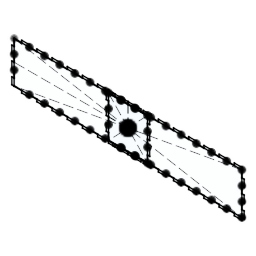
MVP (Autodesk Fusion 360 design; units mm, degrees)
part number: 2026-03-07-18-20-50-739
Autodesk Fusion 360 part; units mm, degrees
sketch "Front" plane through (0, 0, 0) normal (0, 0, 1) x (1, 0, 0)
  line L0 (132, 16) -> (-132, 16)
  line L1 (-132, 16) -> (-132, -16)
  line L2 (-132, -16) -> (132, -16)
  line L3 (132, -16) -> (132, 16)
  line L4 (132, 16) -> (-132, -16) construction
  line L5 (-132, 16) -> (132, -16) construction
  line L6 (152, 26) -> (-152, 26)
  line L7 (-152, 26) -> (-152, -26)
  line L8 (-152, -26) -> (152, -26)
  line L9 (152, -26) -> (152, 26)
  line L10 (152, 26) -> (-152, -26) construction
  line L11 (-152, 26) -> (152, -26) construction
  line L12 (0, 0) -> (0, -16) construction
  line L13 (0, 0) -> (12, 0) construction
  line L14 (0, 0) -> (-132, 0) construction
  line L15 (-132, 0) -> (-132, -19) construction
  line L16 (-132, -19) -> (-136, -19) construction
  line L17 (-136, -19) -> (-148, -19) construction
  line L18 (-142, -19) -> (-142, -14.5) construction
  circle A0 centre (-142, -14.5) radius 1.5
  circle A1 centre (-142, 14.5) radius 1.5
  circle A2 centre (142, 14.5) radius 1.5
  circle A3 centre (142, -14.5) radius 1.5
  line L19 (-152, 26) -> (-152, 29)
  line L20 (-152, 29) -> (-141.8667, 29)
  line L21 (-141.8667, 29) -> (-141.8667, 26)
  line L22 (-141.8667, 26) -> (-131.7333, 26)
  line L23 (-121.6, 29) -> (-121.6, 26)
  line L24 (-121.6, 26) -> (-111.4667, 26)
  line L25 (-131.7333, 29) -> (-121.6, 29)
  line L26 (-131.7333, 26) -> (-131.7333, 29)
  line L27 (-101.3333, 29) -> (-101.3333, 26)
  line L28 (-101.3333, 26) -> (-91.2, 26)
  line L29 (-111.4667, 29) -> (-101.3333, 29)
  line L30 (-111.4667, 26) -> (-111.4667, 29)
  line L31 (-81.0667, 29) -> (-81.0667, 26)
  line L32 (-81.0667, 26) -> (-70.9333, 26)
  line L33 (-91.2, 29) -> (-81.0667, 29)
  line L34 (-91.2, 26) -> (-91.2, 29)
  line L35 (-60.8, 29) -> (-60.8, 26)
  line L36 (-60.8, 26) -> (-50.6667, 26)
  line L37 (-70.9333, 29) -> (-60.8, 29)
  line L38 (-70.9333, 26) -> (-70.9333, 29)
  line L39 (-40.5333, 29) -> (-40.5333, 26)
  line L40 (-40.5333, 26) -> (-30.4, 26)
  line L41 (-50.6667, 29) -> (-40.5333, 29)
  line L42 (-50.6667, 26) -> (-50.6667, 29)
  line L43 (-20.2667, 29) -> (-20.2667, 26)
  line L44 (-20.2667, 26) -> (-10.1333, 26)
  line L45 (-30.4, 29) -> (-20.2667, 29)
  line L46 (-30.4, 26) -> (-30.4, 29)
  line L47 (0, 29) -> (0, 26)
  line L48 (0, 26) -> (10.1333, 26)
  line L49 (-10.1333, 29) -> (0, 29)
  line L50 (-10.1333, 26) -> (-10.1333, 29)
  line L51 (20.2667, 29) -> (20.2667, 26)
  line L52 (20.2667, 26) -> (30.4, 26)
  line L53 (10.1333, 29) -> (20.2667, 29)
  line L54 (10.1333, 26) -> (10.1333, 29)
  line L55 (40.5333, 29) -> (40.5333, 26)
  line L56 (40.5333, 26) -> (50.6667, 26)
  line L57 (30.4, 29) -> (40.5333, 29)
  line L58 (30.4, 26) -> (30.4, 29)
  line L59 (60.8, 29) -> (60.8, 26)
  line L60 (60.8, 26) -> (70.9333, 26)
  line L61 (50.6667, 29) -> (60.8, 29)
  line L62 (50.6667, 26) -> (50.6667, 29)
  line L63 (81.0667, 29) -> (81.0667, 26)
  line L64 (81.0667, 26) -> (91.2, 26)
  line L65 (70.9333, 29) -> (81.0667, 29)
  line L66 (70.9333, 26) -> (70.9333, 29)
  line L67 (101.3333, 29) -> (101.3333, 26)
  line L68 (101.3333, 26) -> (111.4667, 26)
  line L69 (91.2, 29) -> (101.3333, 29)
  line L70 (91.2, 26) -> (91.2, 29)
  line L71 (121.6, 29) -> (121.6, 26)
  line L72 (121.6, 26) -> (131.7333, 26)
  line L73 (111.4667, 29) -> (121.6, 29)
  line L74 (111.4667, 26) -> (111.4667, 29)
  line L75 (141.8667, 29) -> (141.8667, 26)
  line L76 (141.8667, 26) -> (152, 26)
  line L77 (131.7333, 29) -> (141.8667, 29)
  line L78 (131.7333, 26) -> (131.7333, 29)
  line L79 (-152, -26) -> (-152, -29)
  line L80 (-152, -29) -> (-141.8667, -29)
  line L81 (-141.8667, -29) -> (-141.8667, -26)
  line L82 (-141.8667, -26) -> (-131.7333, -26)
  line L83 (-131.7333, -26) -> (-131.7333, -29)
  line L84 (-131.7333, -29) -> (-121.6, -29)
  line L85 (-121.6, -29) -> (-121.6, -26)
  line L86 (-121.6, -26) -> (-111.4667, -26)
  line L87 (-111.4667, -26) -> (-111.4667, -29)
  line L88 (-111.4667, -29) -> (-101.3333, -29)
  line L89 (-101.3333, -29) -> (-101.3333, -26)
  line L90 (-101.3333, -26) -> (-91.2, -26)
  line L91 (-91.2, -26) -> (-91.2, -29)
  line L92 (-91.2, -29) -> (-81.0667, -29)
  line L93 (-81.0667, -29) -> (-81.0667, -26)
  line L94 (-81.0667, -26) -> (-70.9333, -26)
  line L95 (-70.9333, -26) -> (-70.9333, -29)
  line L96 (-70.9333, -29) -> (-60.8, -29)
  line L97 (-60.8, -29) -> (-60.8, -26)
  line L98 (-60.8, -26) -> (-50.6667, -26)
  line L99 (-50.6667, -26) -> (-50.6667, -29)
  line L100 (-50.6667, -29) -> (-40.5333, -29)
  line L101 (-40.5333, -29) -> (-40.5333, -26)
  line L102 (-40.5333, -26) -> (-30.4, -26)
  line L103 (-30.4, -26) -> (-30.4, -29)
  line L104 (-30.4, -29) -> (-20.2667, -29)
  line L105 (-20.2667, -29) -> (-20.2667, -26)
  line L106 (-20.2667, -26) -> (-10.1333, -26)
  line L107 (-10.1333, -26) -> (-10.1333, -29)
  line L108 (-10.1333, -29) -> (0, -29)
  line L109 (0, -29) -> (0, -26)
  line L110 (0, -26) -> (10.1333, -26)
  line L111 (10.1333, -26) -> (10.1333, -29)
  line L112 (10.1333, -29) -> (20.2667, -29)
  line L113 (20.2667, -29) -> (20.2667, -26)
  line L114 (20.2667, -26) -> (30.4, -26)
  line L115 (30.4, -26) -> (30.4, -29)
  line L116 (30.4, -29) -> (40.5333, -29)
  line L117 (40.5333, -29) -> (40.5333, -26)
  line L118 (40.5333, -26) -> (50.6667, -26)
  line L119 (50.6667, -26) -> (50.6667, -29)
  line L120 (50.6667, -29) -> (60.8, -29)
  line L121 (60.8, -29) -> (60.8, -26)
  line L122 (60.8, -26) -> (70.9333, -26)
  line L123 (70.9333, -26) -> (70.9333, -29)
  line L124 (70.9333, -29) -> (81.0667, -29)
  line L125 (81.0667, -29) -> (81.0667, -26)
  line L126 (81.0667, -26) -> (91.2, -26)
  line L127 (91.2, -26) -> (91.2, -29)
  line L128 (91.2, -29) -> (101.3333, -29)
  line L129 (101.3333, -29) -> (101.3333, -26)
  line L130 (101.3333, -26) -> (111.4667, -26)
  line L131 (111.4667, -26) -> (111.4667, -29)
  line L132 (111.4667, -29) -> (121.6, -29)
  line L133 (121.6, -29) -> (121.6, -26)
  line L134 (121.6, -26) -> (131.7333, -26)
  line L135 (131.7333, -26) -> (131.7333, -29)
  line L136 (131.7333, -29) -> (141.8667, -29)
  line L137 (141.8667, -29) -> (141.8667, -26)
  line L138 (141.8667, -26) -> (152, -26)
  line L139 (-152, -26) -> (-152, -17.3333)
  line L140 (-152, -17.3333) -> (-155, -17.3333)
  line L141 (-155, -17.3333) -> (-155, -8.6667)
  line L142 (-155, -8.6667) -> (-152, -8.6667)
  line L143 (-155, 0) -> (-155, 8.6667)
  line L144 (-152, 0) -> (-155, 0)
  line L145 (-155, 8.6667) -> (-152, 8.6667)
  line L146 (-152, -8.6667) -> (-152, 0)
  line L147 (-155, 17.3333) -> (-155, 26)
  line L148 (-152, 17.3333) -> (-155, 17.3333)
  line L149 (-155, 26) -> (-152, 26)
  line L150 (-152, 8.6667) -> (-152, 17.3333)
  line L151 (155, 17.3333) -> (155, 26)
  line L152 (152, 17.3333) -> (155, 17.3333)
  line L153 (152, 8.6667) -> (152, 17.3333)
  line L154 (155, 26) -> (152, 26)
  line L155 (155, 8.6667) -> (152, 8.6667)
  line L156 (155, 0) -> (155, 8.6667)
  line L157 (152, 0) -> (155, 0)
  line L158 (152, -8.6667) -> (152, 0)
  line L159 (155, -17.3333) -> (155, -8.6667)
  line L160 (152, -17.3333) -> (155, -17.3333)
  line L161 (152, -26) -> (152, -17.3333)
  line L162 (155, -8.6667) -> (152, -8.6667)
  dimension "d15" = 264
  dimension "d16" = 32
  dimension "d17" = 304
  dimension "d18" = 52
  dimension "d58" = 16
  dimension "d63" = 12
  dimension "d71" = 132
  dimension "d72" = 19
  dimension "d73" = 4
  dimension "d74" = 12
  dimension "d75" = 4.5
  dimension "d76" = 3
  dimension "d86" = 3
  dimension "d87" = 10.1333
  dimension "d88" = 3
  dimension "d89" = 10.1333
  dimension "d92" = 283.7333
  dimension "d93" = 0
  dimension "d94" = 3
  dimension "d95" = 10.1333
  dimension "d96" = 3
  dimension "d97" = 10.1333
  dimension "d100" = 283.7333
  dimension "d101" = 0
  dimension "d105" = 8.6667
  dimension "d106" = 3
  dimension "d107" = 8.6667
  dimension "d108" = 3
  dimension "d111" = 0
  dimension "d112" = 34.6667
  constraint horizontal L0
  constraint perpendicular L0 L1
  constraint parallel L0 L2
  constraint parallel L1 L3
  constraint coincident L4 L12.start
  constraint coincident L5 L12.start
  constraint coincident L12.start L13.start
  constraint horizontal L6
  constraint perpendicular L6 L7
  constraint parallel L6 L8
  constraint parallel L7 L9
  constraint coincident L10 L12.start
  constraint coincident L11 L12.start
  constraint perpendicular L2 L12
  constraint horizontal L13
  constraint parallel L0 L14
  constraint perpendicular L2 L15
  constraint perpendicular L15 L16
  constraint parallel L16 L17
  constraint midpoint L17 L18.start
  constraint perpendicular L17 L18
  constraint coincident L18.end A0.centre
  constraint symmetric L14 A0 A1
  constraint symmetric L12 A0 A3
  constraint symmetric L12 A1 A2
  constraint perpendicular L6 L19
  constraint perpendicular L19 L20
  constraint perpendicular L20 L21
  constraint perpendicular L21 L22
  constraint perpendicular L8 L79
  constraint perpendicular L79 L80
  constraint perpendicular L8 L81
  constraint perpendicular L81 L82
  constraint perpendicular L8 L139
  constraint perpendicular L7 L140
  constraint perpendicular L140 L141
  constraint coincident L7 L142.end
  constraint perpendicular L7 L142
  constraint symmetric L7.end L12 L8.end
  constraint symmetric L12 L139.end L160.start
  constraint symmetric L12 L140.end L159.start
  constraint symmetric L12 L141.end L159.end
  constraint symmetric L12 L142.end L158.start
  constraint symmetric L12 L143.start L156.start
  constraint symmetric L12 L143.end L155.start
  constraint symmetric L12 L144.start L157.start
  constraint symmetric L12 L145.end L153.start
  constraint symmetric L12 L147.start L151.start
  constraint symmetric L12 L147.end L151.end
  constraint symmetric L12 L148.start L152.start
  constraint symmetric L12 L6.end L6.start
  measures "d15" distance of L1.end L2.end
  measures "d16" distance of L0.end L1.end
  measures "d17" distance of L7.end L8.end
  measures "d18" distance of L6.end L7.end
  measures "d58" distance of L12.start L12.end
  measures "d63" distance of L12.start L13.end
  measures "d71" distance of L12.start L14.end
  measures "d72" distance of L14.end L15.end
  measures "d73" distance of L15.end L16.end
  measures "d74" distance of L16.end L17.end
  measures "d75" distance of L18.start L18.end
  measures "d76" diameter of A0
  measures "d86" distance of L6.end L19.end
  measures "d87" distance of L19.end L20.end
  measures "d88" distance of L20.end L21.end
  measures "d89" distance of L21.end L22.end
  measures "d94" distance of L7.end L79.end
  measures "d95" distance of L79.end L80.end
  measures "d96" distance of L80.end L81.end
  measures "d97" distance of L81.end L82.end
  measures "d105" distance of L7.end L139.end
  measures "d106" distance of L139.end L140.end
  measures "d107" distance of L140.end L141.end
  measures "d108" distance of L141.end L142.end
sketch "Clamp base" plane through (0, 0, 0) normal (0, 0, 1) x (1, 0, 0)
  line L0 (6, 19) -> (-6, 19)
  line L1 (-6, 19) -> (-6, -19)
  line L2 (-6, -19) -> (6, -19)
  line L3 (6, -19) -> (6, 19)
  line L4 (6, 19) -> (-6, -19) construction
  line L5 (-6, 19) -> (6, -19) construction
  line L6 (0, 19) -> (0, 14.5) construction
  circle A0 centre (0, 14.5) radius 1.5
  line L7 (0, 0) -> (6, 0) construction
  circle A1 centre (0, -14.5) radius 1.5
  line L8 (0, -19) -> (0, -14.5) construction
  line L9 (6, 19) -> (9, 19)
  line L10 (9, 19) -> (9, -19)
  line L11 (9, -19) -> (6, -19)
  line L12 (6, -19) -> (6, 19)
  line L13 (6, 19) -> (6, 10) construction
  line L14 (6, 10) -> (-6, 10)
  line L15 (6, -10) -> (-6, -10)
  dimension "d19" = 12
  dimension "d20" = 38
  dimension "d21" = 4.5
  dimension "d22" = 3
  dimension "d23" = 3
  dimension "d24" = 38
  dimension "d67" = 9
  dimension "d68" = 12
  constraint horizontal L0
  constraint perpendicular L0 L1
  constraint parallel L0 L2
  constraint parallel L1 L3
  constraint coincident L4 L7.start
  constraint coincident L5 L7.start
  constraint coincident L7.start origin
  constraint midpoint L0 L6.start
  constraint perpendicular L0 L6
  constraint coincident L6.end A0.centre
  constraint midpoint L3 L7.end
  constraint symmetric L6.start L7 L8.start
  constraint symmetric L6.end L7 A1.centre
  constraint symmetric A0 L7 A1
  constraint horizontal L9
  constraint vertical L10
  constraint horizontal L11
  constraint vertical L12
  constraint perpendicular L0 L13
  constraint perpendicular L1 L14
  constraint symmetric L7 L13.end L15.start
  constraint symmetric L7 L14.end L15.end
  measures "d19" distance of L1.end L2.end
  measures "d20" distance of L0.end L1.end
  measures "d21" distance of L6.start L6.end
  measures "d22" diameter of A0
  measures "d23" distance of L0.start L9.end
  measures "d24" distance of L0.start L2.end
  measures "d67" distance of L0.start L13.end
  measures "d68" distance of L13.end L14.end
extrude "Extrude3" add sketch "Clamp base" along normal blind 2 contours L0 L1 L3 L12 L14 | L1 L3 L12 L14 L15 | L1 L2 L3 L12 L15
extrude "Extrude4" add sketch "Clamp base" along normal blind 11.5 contours L3 L9 L10 L11 L12
sketch "Clamp support wall" plane through (9, 0, 0) normal (1, 0, 0) x (0, 0, -1)
  line L0 (0, -19) -> (0, 19)
  line L1 (0, 19) -> (-11.5, 19)
  line L2 (-11.5, 19) -> (-11.5, -19)
  line L3 (-11.5, -19) -> (0, -19)
  line L4 (-11.5, 19) -> (-5.75, 19) construction
  line L5 (-5.75, 19) -> (-5.75, 17) construction
  line L6 (0, 0) -> (-2, 0) construction
  line L7 (-11.5, 19) -> (-6.1, 19)
  line L8 (-11.5, 19) -> (-6.1, 19)
  line L9 (-6.1, 19) -> (-6.1, 7)
  line L10 (-6.1, 7) -> (-11.5, 7)
  line L11 (-11.5, 7) -> (-11.5, 19)
  line L12 (-6.1, -7) -> (-11.5, -7)
  line L13 (-11.5, -7) -> (-11.5, -19)
  line L14 (-11.5, -19) -> (-6.1, -19)
  line L15 (-6.1, -19) -> (-6.1, -7)
  line L16 (0, 19) -> (0, 10) construction
  line L17 (0, 10) -> (-6.1, 10)
  line L18 (0, -10) -> (-6.1, -10)
  line L19 (-6.1, 7) -> (-6.1, -7)
  dimension "d42" = 2
  dimension "d43" = 2
  dimension "d44" = 5.4
  dimension "d45" = 5.4
  dimension "d46" = 12
  dimension "d77" = 9
  constraint coincident L1.end L2.start
  constraint midpoint L1 L4.end
  constraint perpendicular L1 L5
  constraint coincident L6.start origin
  constraint perpendicular L0 L6
  constraint perpendicular L5 L7
  constraint horizontal L8
  constraint vertical L9
  constraint horizontal L10
  constraint vertical L11
  constraint symmetric L6 L1.end L2.end
  constraint symmetric L6 L7.end L14.end
  constraint symmetric L6 L9.end L12.start
  constraint symmetric L6 L10.end L12.end
  constraint coincident L0.end L1.start
  constraint perpendicular L1 L16
  constraint coincident L9 L17.end
  constraint perpendicular L9 L17
  constraint symmetric L6 L16.end L18.start
  constraint symmetric L6 L17.end L18.end
  measures "d42" distance of L4.end L5.end
  measures "d43" distance of L6.start L6.end
  measures "d44" distance of L1.end L7.end
  measures "d45" distance of L1.end L7.end
  measures "d46" distance of L1.end L10.end
  measures "d77" distance of L0.end L16.end
extrude "Extrude5" add sketch "Clamp support wall" along normal blind 5 contours L2 L3 L12 L13 L14 L15 | L1 L2 L7 L8 L9 L10 L11
sketch "Clamp grooves" plane through (14, 0, 0) normal (1, 0, 0) x (0, 0, -1)
  line L0 (-11.5, 7) -> (-6.1, 7)
  line L1 (-6.1, 7) -> (-6.1, 19)
  line L2 (-6.1, 19) -> (-11.5, 19)
  line L3 (-11.5, 19) -> (-11.5, 7)
  line L4 (0, 0) -> (-2, 0) construction
  line L5 (-6.1, 7) -> (-8.1, 7)
  line L6 (-8.1, 7) -> (-8.1, 17)
  line L7 (-8.1, 17) -> (-9.5, 17)
  line L8 (-9.5, 17) -> (-9.5, 7)
  line L9 (-8.1, -7) -> (-8.1, -17)
  line L10 (-8.1, -17) -> (-9.5, -17)
  line L11 (-9.5, -17) -> (-9.5, -7)
  line L12 (-9.5, 7) -> (-8.1, 7)
  line L13 (-8.1, -7) -> (-9.5, -7)
  dimension "d49" = 2
  dimension "d50" = 2
  dimension "d51" = 10
  dimension "d52" = 1.4
  dimension "d53" = 10
  constraint coincident L4.start origin
  constraint horizontal L4
  constraint coincident L0.end L1.start
  constraint coincident L0 L5.end
  constraint perpendicular L0 L6
  constraint perpendicular L6 L7
  constraint perpendicular L0 L8
  constraint symmetric L4 L5.end L9.start
  constraint symmetric L4 L6.end L9.end
  constraint symmetric L4 L7.end L10.end
  constraint symmetric L4 L8.end L11.end
  measures "d49" distance of L4.start L4.end
  measures "d50" distance of L0.end L5.end
  measures "d51" distance of L5.end L6.end
  measures "d52" distance of L6.end L7.end
  measures "d53" distance of L7.end L8.end
extrude "Extrude8" cut sketch "Clamp grooves" against normal blind 5 contours L0 L6 L7 L8 L12 | L9 L10 L11 L13
extrude "Extrude9" cut sketch "Clamp base" along normal blind 2 contours L1 L3 L12 L14 L15
extrude "Extrude10" cut sketch "Clamp support wall" against normal blind 3 contours L0 L9 L15 L17 L18 L19
sketch "Back" plane through (0, 0, 0) normal (0, 0, 1) x (1, 0, 0)
  line L0 (152, 26) -> (-152, 26)
  line L1 (-152, 26) -> (-152, -26)
  line L2 (-152, -26) -> (152, -26)
  line L3 (152, -26) -> (152, 26)
  line L4 (152, 26) -> (-152, -26) construction
  line L5 (-152, 26) -> (152, -26) construction
  line L6 (0, 0) -> (0, 26) construction
  line L7 (0, 0) -> (-152, 0) construction
  line L8 (-152, 26) -> (-152, 29)
  line L9 (-152, 29) -> (-141.8667, 29)
  line L10 (-141.8667, 29) -> (-141.8667, 26)
  line L11 (-141.8667, 26) -> (-131.7333, 26)
  line L12 (-131.7333, 29) -> (-121.6, 29)
  line L13 (-121.6, 29) -> (-121.6, 26)
  line L14 (-121.6, 26) -> (-111.4667, 26)
  line L15 (-131.7333, 26) -> (-131.7333, 29)
  line L16 (-111.4667, 29) -> (-101.3333, 29)
  line L17 (-101.3333, 29) -> (-101.3333, 26)
  line L18 (-101.3333, 26) -> (-91.2, 26)
  line L19 (-111.4667, 26) -> (-111.4667, 29)
  line L20 (-91.2, 29) -> (-81.0667, 29)
  line L21 (-81.0667, 29) -> (-81.0667, 26)
  line L22 (-81.0667, 26) -> (-70.9333, 26)
  line L23 (-91.2, 26) -> (-91.2, 29)
  line L24 (-70.9333, 29) -> (-60.8, 29)
  line L25 (-60.8, 29) -> (-60.8, 26)
  line L26 (-60.8, 26) -> (-50.6667, 26)
  line L27 (-70.9333, 26) -> (-70.9333, 29)
  line L28 (-50.6667, 29) -> (-40.5333, 29)
  line L29 (-40.5333, 29) -> (-40.5333, 26)
  line L30 (-40.5333, 26) -> (-30.4, 26)
  line L31 (-50.6667, 26) -> (-50.6667, 29)
  line L32 (-30.4, 29) -> (-20.2667, 29)
  line L33 (-20.2667, 29) -> (-20.2667, 26)
  line L34 (-20.2667, 26) -> (-10.1333, 26)
  line L35 (-30.4, 26) -> (-30.4, 29)
  line L36 (-10.1333, 29) -> (0, 29)
  line L37 (0, 29) -> (0, 26)
  line L38 (0, 26) -> (10.1333, 26)
  line L39 (-10.1333, 26) -> (-10.1333, 29)
  line L40 (10.1333, 29) -> (20.2667, 29)
  line L41 (20.2667, 29) -> (20.2667, 26)
  line L42 (20.2667, 26) -> (30.4, 26)
  line L43 (10.1333, 26) -> (10.1333, 29)
  line L44 (30.4, 29) -> (40.5333, 29)
  line L45 (40.5333, 29) -> (40.5333, 26)
  line L46 (40.5333, 26) -> (50.6667, 26)
  line L47 (30.4, 26) -> (30.4, 29)
  line L48 (50.6667, 29) -> (60.8, 29)
  line L49 (60.8, 29) -> (60.8, 26)
  line L50 (60.8, 26) -> (70.9333, 26)
  line L51 (50.6667, 26) -> (50.6667, 29)
  line L52 (70.9333, 29) -> (81.0667, 29)
  line L53 (81.0667, 29) -> (81.0667, 26)
  line L54 (81.0667, 26) -> (91.2, 26)
  line L55 (70.9333, 26) -> (70.9333, 29)
  line L56 (91.2, 29) -> (101.3333, 29)
  line L57 (101.3333, 29) -> (101.3333, 26)
  line L58 (101.3333, 26) -> (111.4667, 26)
  line L59 (91.2, 26) -> (91.2, 29)
  line L60 (111.4667, 29) -> (121.6, 29)
  line L61 (121.6, 29) -> (121.6, 26)
  line L62 (121.6, 26) -> (131.7333, 26)
  line L63 (111.4667, 26) -> (111.4667, 29)
  line L64 (131.7333, 29) -> (141.8667, 29)
  line L65 (141.8667, 29) -> (141.8667, 26)
  line L66 (141.8667, 26) -> (152, 26)
  line L67 (131.7333, 26) -> (131.7333, 29)
  line L68 (-152, -29) -> (-141.8667, -29)
  line L69 (-141.8667, -29) -> (-141.8667, -26)
  line L70 (-141.8667, -26) -> (-131.7333, -26)
  line L71 (-152, -26) -> (-152, -29)
  line L72 (-131.7333, -29) -> (-121.6, -29)
  line L73 (-131.7333, -26) -> (-131.7333, -29)
  line L74 (-121.6, -29) -> (-121.6, -26)
  line L75 (-121.6, -26) -> (-111.4667, -26)
  line L76 (-111.4667, -29) -> (-101.3333, -29)
  line L77 (-111.4667, -26) -> (-111.4667, -29)
  line L78 (-101.3333, -29) -> (-101.3333, -26)
  line L79 (-101.3333, -26) -> (-91.2, -26)
  line L80 (-91.2, -29) -> (-81.0667, -29)
  line L81 (-91.2, -26) -> (-91.2, -29)
  line L82 (-81.0667, -29) -> (-81.0667, -26)
  line L83 (-81.0667, -26) -> (-70.9333, -26)
  line L84 (-70.9333, -29) -> (-60.8, -29)
  line L85 (-70.9333, -26) -> (-70.9333, -29)
  line L86 (-60.8, -29) -> (-60.8, -26)
  line L87 (-60.8, -26) -> (-50.6667, -26)
  line L88 (-50.6667, -29) -> (-40.5333, -29)
  line L89 (-50.6667, -26) -> (-50.6667, -29)
  line L90 (-40.5333, -29) -> (-40.5333, -26)
  line L91 (-40.5333, -26) -> (-30.4, -26)
  line L92 (-30.4, -29) -> (-20.2667, -29)
  line L93 (-30.4, -26) -> (-30.4, -29)
  line L94 (-20.2667, -29) -> (-20.2667, -26)
  line L95 (-20.2667, -26) -> (-10.1333, -26)
  line L96 (-10.1333, -29) -> (0, -29)
  line L97 (-10.1333, -26) -> (-10.1333, -29)
  line L98 (0, -29) -> (0, -26)
  line L99 (0, -26) -> (10.1333, -26)
  line L100 (10.1333, -29) -> (20.2667, -29)
  line L101 (10.1333, -26) -> (10.1333, -29)
  line L102 (20.2667, -29) -> (20.2667, -26)
  line L103 (20.2667, -26) -> (30.4, -26)
  line L104 (30.4, -29) -> (40.5333, -29)
  line L105 (30.4, -26) -> (30.4, -29)
  line L106 (40.5333, -29) -> (40.5333, -26)
  line L107 (40.5333, -26) -> (50.6667, -26)
  line L108 (50.6667, -29) -> (60.8, -29)
  line L109 (50.6667, -26) -> (50.6667, -29)
  line L110 (60.8, -29) -> (60.8, -26)
  line L111 (60.8, -26) -> (70.9333, -26)
  line L112 (70.9333, -29) -> (81.0667, -29)
  line L113 (70.9333, -26) -> (70.9333, -29)
  line L114 (81.0667, -29) -> (81.0667, -26)
  line L115 (81.0667, -26) -> (91.2, -26)
  line L116 (91.2, -29) -> (101.3333, -29)
  line L117 (91.2, -26) -> (91.2, -29)
  line L118 (101.3333, -29) -> (101.3333, -26)
  line L119 (101.3333, -26) -> (111.4667, -26)
  line L120 (111.4667, -29) -> (121.6, -29)
  line L121 (111.4667, -26) -> (111.4667, -29)
  line L122 (121.6, -29) -> (121.6, -26)
  line L123 (121.6, -26) -> (131.7333, -26)
  line L124 (131.7333, -29) -> (141.8667, -29)
  line L125 (131.7333, -26) -> (131.7333, -29)
  line L126 (141.8667, -29) -> (141.8667, -26)
  line L127 (141.8667, -26) -> (152, -26)
  line L128 (-152, -26) -> (-152, -17.3333)
  line L129 (-152, -17.3333) -> (-155, -17.3333)
  line L130 (-155, -17.3333) -> (-155, -8.6667)
  line L131 (-155, -8.6667) -> (-152, -8.6667)
  line L132 (152, -26) -> (152, -17.3333)
  line L133 (152, -17.3333) -> (155, -17.3333)
  line L134 (155, -8.6667) -> (152, -8.6667)
  line L135 (155, -17.3333) -> (155, -8.6667)
  line L136 (-152, -8.6667) -> (-152, 0)
  line L137 (-152, 0) -> (-155, 0)
  line L138 (-155, 0) -> (-155, 8.6667)
  line L139 (-155, 8.6667) -> (-152, 8.6667)
  line L140 (-152, 8.6667) -> (-152, 17.3333)
  line L141 (-152, 17.3333) -> (-155, 17.3333)
  line L142 (-155, 17.3333) -> (-155, 26)
  line L143 (-155, 26) -> (-152, 26)
  line L144 (152, 0) -> (155, 0)
  line L145 (155, 0) -> (155, 8.6667)
  line L146 (155, 8.6667) -> (152, 8.6667)
  line L147 (152, -8.6667) -> (152, 0)
  line L148 (152, 17.3333) -> (155, 17.3333)
  line L149 (155, 17.3333) -> (155, 26)
  line L150 (155, 26) -> (152, 26)
  line L151 (152, 8.6667) -> (152, 17.3333)
  line L152 (0, 0) -> (76, 0) construction
  line L153 (81.5, 4) -> (70.5, 4)
  line L154 (70.5, 4) -> (70.5, -4)
  line L155 (70.5, -4) -> (81.5, -4)
  line L156 (81.5, -4) -> (81.5, 4)
  line L157 (81.5, 4) -> (70.5, -4) construction
  line L158 (70.5, 4) -> (81.5, -4) construction
  line L159 (25.5, 11.5) -> (-25.5, 11.5) construction
  line L160 (-25.5, 11.5) -> (-25.5, -11.5) construction
  line L161 (-25.5, -11.5) -> (25.5, -11.5) construction
  line L162 (25.5, -11.5) -> (25.5, 11.5) construction
  line L163 (25.5, 11.5) -> (-25.5, -11.5) construction
  line L164 (-25.5, 11.5) -> (25.5, -11.5) construction
  circle A0 centre (25.5, 11.5) radius 1.5
  circle A1 centre (25.5, -11.5) radius 1.5
  circle A2 centre (-25.5, 11.5) radius 1.5
  circle A3 centre (-25.5, -11.5) radius 1.5
  point P0 (76, 0)
  dimension "d113" = 304
  dimension "d114" = 52
  dimension "d115" = 26
  dimension "d116" = 3
  dimension "d117" = 10.1333
  dimension "d118" = 3
  dimension "d119" = 10.1333
  dimension "d122" = 283.7333
  dimension "d123" = 0
  dimension "d126" = 283.7333
  dimension "d127" = 0
  dimension "d128" = 8.6667
  dimension "d129" = 3
  dimension "d130" = 8.6667
  dimension "d131" = 3
  dimension "d134" = 0
  dimension "d135" = 34.6667
  dimension "d138" = 0
  dimension "d139" = 34.6667
  dimension "d140" = 76
  dimension "d141" = 11
  dimension "d142" = 8
  dimension "d145" = 51
  dimension "d146" = 23
  dimension "d147" = 3
  constraint horizontal L0
  constraint perpendicular L0 L1
  constraint parallel L0 L2
  constraint parallel L1 L3
  constraint coincident L4 L6.start
  constraint coincident L5 L6.start
  constraint coincident L6.start L7.start
  constraint vertical L6
  constraint midpoint L1 L7.end
  constraint perpendicular L0 L8
  constraint perpendicular L8 L9
  constraint perpendicular L0 L10
  constraint perpendicular L10 L11
  constraint symmetric L0.end L7 L1.end
  constraint symmetric L7 L8.end L68.start
  constraint symmetric L7 L9.end L68.end
  constraint symmetric L7 L10.end L69.end
  constraint symmetric L7 L11.end L70.end
  constraint perpendicular L2 L128
  constraint perpendicular L128 L129
  constraint perpendicular L129 L130
  constraint perpendicular L1 L131
  constraint symmetric L6 L1.end L2.end
  constraint symmetric L6 L128.end L132.end
  constraint symmetric L6 L129.end L133.end
  constraint symmetric L6 L130.end L134.start
  constraint symmetric L6 L131.end L134.end
  constraint perpendicular L149 L152
  constraint horizontal L153
  constraint perpendicular L153 L154
  constraint parallel L153 L155
  constraint parallel L154 L156
  constraint coincident L157 P0
  constraint coincident L158 P0
  constraint coincident P0 L152.end
  constraint horizontal L159
  constraint perpendicular L159 L160
  constraint parallel L159 L161
  constraint parallel L160 L162
  constraint coincident L163 L6.start
  constraint coincident L164 L6.start
  constraint coincident L159.start L162.end
  constraint symmetric L152 A0 A1
  constraint symmetric L6 A0 A2
  constraint symmetric L6 A1 A3
  measures "d113" distance of L1.end L2.end
  measures "d114" distance of L0.end L1.end
  measures "d115" distance of L6.start L6.end
  measures "d116" distance of L0.end L8.end
  measures "d117" distance of L8.end L9.end
  measures "d118" distance of L9.end L10.end
  measures "d119" distance of L10.end L11.end
  measures "d128" distance of L1.end L128.end
  measures "d129" distance of L128.end L129.end
  measures "d130" distance of L129.end L130.end
  measures "d131" distance of L130.end L131.end
  measures "d140" distance of L6.start P0
  measures "d141" distance of L154.end L155.end
  measures "d142" distance of L153.end L154.end
  measures "d145" distance of L160.end L161.end
  measures "d146" distance of L159.end L160.end
  measures "d147" diameter of A0
sketch "Top/Bottom" plane through (0, 0, 0) normal (0, 0, 1) x (1, 0, 0)
  line L0 (152, 27.5) -> (-152, 27.5)
  line L1 (-152, 27.5) -> (-152, -27.5)
  line L2 (-152, -27.5) -> (152, -27.5)
  line L3 (152, -27.5) -> (152, 27.5)
  line L4 (152, 27.5) -> (-152, -27.5) construction
  line L5 (-152, 27.5) -> (152, -27.5) construction
  line L6 (-152, 27.5) -> (-141.8667, 27.5)
  line L7 (-141.8667, 27.5) -> (-141.8667, 30.5)
  line L8 (-141.8667, 30.5) -> (-131.7333, 30.5)
  line L9 (-131.7333, 30.5) -> (-131.7333, 27.5)
  line L10 (0, 0) -> (0, 27.5) construction
  line L11 (0, 0) -> (-152, 0) construction
  line L12 (-152, -27.5) -> (-141.8667, -27.5)
  line L13 (-141.8667, -27.5) -> (-141.8667, -30.5)
  line L14 (-141.8667, -30.5) -> (-131.7333, -30.5)
  line L15 (-131.7333, -30.5) -> (-131.7333, -27.5)
  line L16 (-111.4667, 30.5) -> (-111.4667, 27.5)
  line L17 (-121.6, 30.5) -> (-111.4667, 30.5)
  line L18 (-121.6, 27.5) -> (-121.6, 30.5)
  line L19 (-131.7333, 27.5) -> (-121.6, 27.5)
  line L20 (-91.2, 30.5) -> (-91.2, 27.5)
  line L21 (-101.3333, 30.5) -> (-91.2, 30.5)
  line L22 (-101.3333, 27.5) -> (-101.3333, 30.5)
  line L23 (-111.4667, 27.5) -> (-101.3333, 27.5)
  line L24 (-70.9333, 30.5) -> (-70.9333, 27.5)
  line L25 (-81.0667, 30.5) -> (-70.9333, 30.5)
  line L26 (-81.0667, 27.5) -> (-81.0667, 30.5)
  line L27 (-91.2, 27.5) -> (-81.0667, 27.5)
  line L28 (-50.6667, 30.5) -> (-50.6667, 27.5)
  line L29 (-60.8, 30.5) -> (-50.6667, 30.5)
  line L30 (-60.8, 27.5) -> (-60.8, 30.5)
  line L31 (-70.9333, 27.5) -> (-60.8, 27.5)
  line L32 (-30.4, 30.5) -> (-30.4, 27.5)
  line L33 (-40.5333, 30.5) -> (-30.4, 30.5)
  line L34 (-40.5333, 27.5) -> (-40.5333, 30.5)
  line L35 (-50.6667, 27.5) -> (-40.5333, 27.5)
  line L36 (-10.1333, 30.5) -> (-10.1333, 27.5)
  line L37 (-20.2667, 30.5) -> (-10.1333, 30.5)
  line L38 (-20.2667, 27.5) -> (-20.2667, 30.5)
  line L39 (-30.4, 27.5) -> (-20.2667, 27.5)
  line L40 (10.1333, 30.5) -> (10.1333, 27.5)
  line L41 (0, 30.5) -> (10.1333, 30.5)
  line L42 (0, 27.5) -> (0, 30.5)
  line L43 (-10.1333, 27.5) -> (0, 27.5)
  line L44 (30.4, 30.5) -> (30.4, 27.5)
  line L45 (20.2667, 30.5) -> (30.4, 30.5)
  line L46 (20.2667, 27.5) -> (20.2667, 30.5)
  line L47 (10.1333, 27.5) -> (20.2667, 27.5)
  line L48 (50.6667, 30.5) -> (50.6667, 27.5)
  line L49 (40.5333, 30.5) -> (50.6667, 30.5)
  line L50 (40.5333, 27.5) -> (40.5333, 30.5)
  line L51 (30.4, 27.5) -> (40.5333, 27.5)
  line L52 (70.9333, 30.5) -> (70.9333, 27.5)
  line L53 (60.8, 30.5) -> (70.9333, 30.5)
  line L54 (60.8, 27.5) -> (60.8, 30.5)
  line L55 (50.6667, 27.5) -> (60.8, 27.5)
  line L56 (91.2, 30.5) -> (91.2, 27.5)
  line L57 (81.0667, 30.5) -> (91.2, 30.5)
  line L58 (81.0667, 27.5) -> (81.0667, 30.5)
  line L59 (70.9333, 27.5) -> (81.0667, 27.5)
  line L60 (111.4667, 30.5) -> (111.4667, 27.5)
  line L61 (101.3333, 30.5) -> (111.4667, 30.5)
  line L62 (101.3333, 27.5) -> (101.3333, 30.5)
  line L63 (91.2, 27.5) -> (101.3333, 27.5)
  line L64 (131.7333, 30.5) -> (131.7333, 27.5)
  line L65 (121.6, 30.5) -> (131.7333, 30.5)
  line L66 (121.6, 27.5) -> (121.6, 30.5)
  line L67 (111.4667, 27.5) -> (121.6, 27.5)
  line L68 (152, 30.5) -> (152, 27.5)
  line L69 (141.8667, 30.5) -> (152, 30.5)
  line L70 (141.8667, 27.5) -> (141.8667, 30.5)
  line L71 (131.7333, 27.5) -> (141.8667, 27.5)
  line L72 (-121.6, -27.5) -> (-121.6, -30.5)
  line L73 (-121.6, -30.5) -> (-111.4667, -30.5)
  line L74 (-111.4667, -30.5) -> (-111.4667, -27.5)
  line L75 (-131.7333, -27.5) -> (-121.6, -27.5)
  line L76 (-101.3333, -27.5) -> (-101.3333, -30.5)
  line L77 (-101.3333, -30.5) -> (-91.2, -30.5)
  line L78 (-91.2, -30.5) -> (-91.2, -27.5)
  line L79 (-111.4667, -27.5) -> (-101.3333, -27.5)
  line L80 (-81.0667, -27.5) -> (-81.0667, -30.5)
  line L81 (-81.0667, -30.5) -> (-70.9333, -30.5)
  line L82 (-70.9333, -30.5) -> (-70.9333, -27.5)
  line L83 (-91.2, -27.5) -> (-81.0667, -27.5)
  line L84 (-60.8, -27.5) -> (-60.8, -30.5)
  line L85 (-60.8, -30.5) -> (-50.6667, -30.5)
  line L86 (-50.6667, -30.5) -> (-50.6667, -27.5)
  line L87 (-70.9333, -27.5) -> (-60.8, -27.5)
  line L88 (-40.5333, -27.5) -> (-40.5333, -30.5)
  line L89 (-40.5333, -30.5) -> (-30.4, -30.5)
  line L90 (-30.4, -30.5) -> (-30.4, -27.5)
  line L91 (-50.6667, -27.5) -> (-40.5333, -27.5)
  line L92 (-20.2667, -27.5) -> (-20.2667, -30.5)
  line L93 (-20.2667, -30.5) -> (-10.1333, -30.5)
  line L94 (-10.1333, -30.5) -> (-10.1333, -27.5)
  line L95 (-30.4, -27.5) -> (-20.2667, -27.5)
  line L96 (0, -27.5) -> (0, -30.5)
  line L97 (0, -30.5) -> (10.1333, -30.5)
  line L98 (10.1333, -30.5) -> (10.1333, -27.5)
  line L99 (-10.1333, -27.5) -> (0, -27.5)
  line L100 (20.2667, -27.5) -> (20.2667, -30.5)
  line L101 (20.2667, -30.5) -> (30.4, -30.5)
  line L102 (30.4, -30.5) -> (30.4, -27.5)
  line L103 (10.1333, -27.5) -> (20.2667, -27.5)
  line L104 (40.5333, -27.5) -> (40.5333, -30.5)
  line L105 (40.5333, -30.5) -> (50.6667, -30.5)
  line L106 (50.6667, -30.5) -> (50.6667, -27.5)
  line L107 (30.4, -27.5) -> (40.5333, -27.5)
  line L108 (60.8, -27.5) -> (60.8, -30.5)
  line L109 (60.8, -30.5) -> (70.9333, -30.5)
  line L110 (70.9333, -30.5) -> (70.9333, -27.5)
  line L111 (50.6667, -27.5) -> (60.8, -27.5)
  line L112 (81.0667, -27.5) -> (81.0667, -30.5)
  line L113 (81.0667, -30.5) -> (91.2, -30.5)
  line L114 (91.2, -30.5) -> (91.2, -27.5)
  line L115 (70.9333, -27.5) -> (81.0667, -27.5)
  line L116 (101.3333, -27.5) -> (101.3333, -30.5)
  line L117 (101.3333, -30.5) -> (111.4667, -30.5)
  line L118 (111.4667, -30.5) -> (111.4667, -27.5)
  line L119 (91.2, -27.5) -> (101.3333, -27.5)
  line L120 (121.6, -27.5) -> (121.6, -30.5)
  line L121 (121.6, -30.5) -> (131.7333, -30.5)
  line L122 (131.7333, -30.5) -> (131.7333, -27.5)
  line L123 (111.4667, -27.5) -> (121.6, -27.5)
  line L124 (141.8667, -27.5) -> (141.8667, -30.5)
  line L125 (141.8667, -30.5) -> (152, -30.5)
  line L126 (152, -30.5) -> (152, -27.5)
  line L127 (131.7333, -27.5) -> (141.8667, -27.5)
  line L128 (-152, -27.5) -> (-155, -27.5)
  line L129 (-155, -27.5) -> (-155, -18.3333)
  line L130 (-155, -18.3333) -> (-152, -18.3333)
  line L131 (-152, -18.3333) -> (-152, -9.1667)
  line L132 (-152, 0) -> (-152, 9.1667)
  line L133 (-155, 0) -> (-152, 0)
  line L134 (-155, -9.1667) -> (-155, 0)
  line L135 (-152, -9.1667) -> (-155, -9.1667)
  line L136 (-152, 18.3333) -> (-152, 27.5)
  line L137 (-155, 18.3333) -> (-152, 18.3333)
  line L138 (-155, 9.1667) -> (-155, 18.3333)
  line L139 (-152, 9.1667) -> (-155, 9.1667)
  line L140 (152, -18.3333) -> (152, -9.1667)
  line L141 (155, -27.5) -> (155, -18.3333)
  line L142 (155, -18.3333) -> (152, -18.3333)
  line L143 (152, -27.5) -> (155, -27.5)
  line L144 (155, -9.1667) -> (155, 0)
  line L145 (155, 0) -> (152, 0)
  line L146 (152, -9.1667) -> (155, -9.1667)
  line L147 (152, 0) -> (152, 9.1667)
  line L148 (155, 9.1667) -> (155, 18.3333)
  line L149 (155, 18.3333) -> (152, 18.3333)
  line L150 (152, 9.1667) -> (155, 9.1667)
  line L151 (152, 18.3333) -> (152, 27.5)
  dimension "d148" = 304
  dimension "d149" = 55
  dimension "d150" = 10.1333
  dimension "d151" = 3
  dimension "d152" = 10.1333
  dimension "d153" = 3
  dimension "d156" = 283.7333
  dimension "d157" = 0
  dimension "d160" = 283.7333
  dimension "d161" = 0
  dimension "d162" = 3
  dimension "d163" = 9.1667
  dimension "d164" = 3
  dimension "d165" = 9.1667
  dimension "d168" = 0
  dimension "d169" = 36.6667
  dimension "d172" = 0
  dimension "d173" = 36.6667
  constraint horizontal L0
  constraint perpendicular L0 L1
  constraint parallel L0 L2
  constraint parallel L1 L3
  constraint coincident L4 L10.start
  constraint coincident L5 L10.start
  constraint coincident L10.start L11.start
  constraint perpendicular L1 L6
  constraint perpendicular L0 L7
  constraint perpendicular L7 L8
  constraint perpendicular L0 L9
  constraint midpoint L0 L10.end
  constraint midpoint L1 L11.end
  constraint symmetric L0.end L11 L1.end
  constraint symmetric L6.end L11 L12.end
  constraint symmetric L7.end L11 L13.end
  constraint symmetric L8.end L11 L14.end
  constraint symmetric L9.end L11 L15.end
  constraint perpendicular L1 L128
  constraint perpendicular L128 L129
  constraint perpendicular L1 L130
  constraint perpendicular L130 L131
  constraint symmetric L10 L1.end L2.end
  constraint symmetric L10 L128.end L141.start
  constraint symmetric L10 L129.end L141.end
  constraint symmetric L10 L130.end L140.start
  constraint symmetric L10 L131.end L140.end
  measures "d148" distance of L1.end L2.end
  measures "d149" distance of L0.end L1.end
  measures "d150" distance of L0.end L6.end
  measures "d151" distance of L6.end L7.end
  measures "d152" distance of L7.end L8.end
  measures "d153" distance of L8.end L9.end
  measures "d162" distance of L1.end L128.end
  measures "d163" distance of L128.end L129.end
  measures "d164" distance of L129.end L130.end
  measures "d165" distance of L130.end L131.end
sketch "Side" plane through (0, 0, 0) normal (0, 0, 1) x (1, 0, 0)
  line L0 (26, 27.5) -> (-26, 27.5)
  line L1 (-26, 27.5) -> (-26, -27.5)
  line L2 (-26, -27.5) -> (26, -27.5)
  line L3 (26, -27.5) -> (26, 27.5)
  line L4 (26, 27.5) -> (-26, -27.5) construction
  line L5 (-26, 27.5) -> (26, -27.5) construction
  line L6 (-26, -27.5) -> (-26, -30.5)
  line L7 (-26, -30.5) -> (-17.3333, -30.5)
  line L8 (-17.3333, -30.5) -> (-17.3333, -27.5)
  line L9 (-17.3333, -27.5) -> (-8.6667, -27.5)
  line L10 (0, -27.5) -> (8.6667, -27.5)
  line L11 (0, -30.5) -> (0, -27.5)
  line L12 (-8.6667, -30.5) -> (0, -30.5)
  line L13 (-8.6667, -27.5) -> (-8.6667, -30.5)
  line L14 (17.3333, -27.5) -> (26, -27.5)
  line L15 (17.3333, -30.5) -> (17.3333, -27.5)
  line L16 (8.6667, -30.5) -> (17.3333, -30.5)
  line L17 (8.6667, -27.5) -> (8.6667, -30.5)
  line L18 (0, 0) -> (0, 27.5) construction
  line L19 (0, 0) -> (-26, 0) construction
  line L20 (-26, 27.5) -> (-26, 30.5)
  line L21 (-26, 30.5) -> (-17.3333, 30.5)
  line L22 (-17.3333, 30.5) -> (-17.3333, 27.5)
  line L23 (-17.3333, 27.5) -> (-8.6667, 27.5)
  line L24 (-8.6667, 30.5) -> (0, 30.5)
  line L25 (0, 30.5) -> (0, 27.5)
  line L26 (0, 27.5) -> (8.6667, 27.5)
  line L27 (-8.6667, 27.5) -> (-8.6667, 30.5)
  line L28 (8.6667, 30.5) -> (17.3333, 30.5)
  line L29 (17.3333, 30.5) -> (17.3333, 27.5)
  line L30 (17.3333, 27.5) -> (26, 27.5)
  line L31 (8.6667, 27.5) -> (8.6667, 30.5)
  line L32 (-26, -27.5) -> (-26, -18.3333)
  line L33 (-26, -18.3333) -> (-29, -18.3333)
  line L34 (-29, -18.3333) -> (-29, -9.1667)
  line L35 (-29, -9.1667) -> (-26, -9.1667)
  line L36 (-29, 9.1667) -> (-26, 9.1667)
  line L37 (-29, 0) -> (-29, 9.1667)
  line L38 (-26, 0) -> (-29, 0)
  line L39 (-26, -9.1667) -> (-26, 0)
  line L40 (-29, 27.5) -> (-26, 27.5)
  line L41 (-29, 18.3333) -> (-29, 27.5)
  line L42 (-26, 18.3333) -> (-29, 18.3333)
  line L43 (-26, 9.1667) -> (-26, 18.3333)
  line L44 (29, -18.3333) -> (29, -9.1667)
  line L45 (29, -9.1667) -> (26, -9.1667)
  line L46 (26, -18.3333) -> (29, -18.3333)
  line L47 (26, -27.5) -> (26, -18.3333)
  line L48 (29, 9.1667) -> (26, 9.1667)
  line L49 (29, 0) -> (29, 9.1667)
  line L50 (26, 0) -> (29, 0)
  line L51 (26, -9.1667) -> (26, 0)
  line L52 (29, 27.5) -> (26, 27.5)
  line L53 (29, 18.3333) -> (29, 27.5)
  line L54 (26, 18.3333) -> (29, 18.3333)
  line L55 (26, 9.1667) -> (26, 18.3333)
  dimension "d174" = 52
  dimension "d175" = 55
  dimension "d176" = 3
  dimension "d177" = 8.6667
  dimension "d178" = 3
  dimension "d179" = 8.6667
  dimension "d182" = 34.6667
  dimension "d183" = 0
  dimension "d186" = 34.6667
  dimension "d187" = 0
  dimension "d188" = 9.1667
  dimension "d189" = 3
  dimension "d190" = 9.1667
  dimension "d191" = 3
  dimension "d194" = 0
  dimension "d195" = 36.6667
  dimension "d198" = 0
  dimension "d199" = 36.6667
  constraint horizontal L0
  constraint perpendicular L0 L1
  constraint parallel L0 L2
  constraint parallel L1 L3
  constraint coincident L4 L18.start
  constraint coincident L5 L18.start
  constraint coincident L18.start L19.start
  constraint perpendicular L2 L6
  constraint perpendicular L6 L7
  constraint perpendicular L2 L8
  constraint perpendicular L8 L9
  constraint midpoint L0 L18.end
  constraint midpoint L1 L19.end
  constraint symmetric L1.end L19 L0.end
  constraint symmetric L6.end L19 L20.end
  constraint symmetric L7.end L19 L21.end
  constraint symmetric L8.end L19 L22.end
  constraint symmetric L9.end L19 L23.end
  constraint perpendicular L2 L32
  constraint perpendicular L32 L33
  constraint perpendicular L33 L34
  constraint perpendicular L1 L35
  constraint symmetric L1.end L18 L2.end
  constraint symmetric L18 L32.end L46.start
  constraint symmetric L18 L33.end L44.start
  constraint symmetric L18 L34.end L44.end
  constraint symmetric L18 L35.end L45.end
  measures "d174" distance of L1.end L2.end
  measures "d175" distance of L0.end L1.end
  measures "d176" distance of L1.end L6.end
  measures "d177" distance of L6.end L7.end
  measures "d178" distance of L7.end L8.end
  measures "d179" distance of L8.end L9.end
  measures "d188" distance of L1.end L32.end
  measures "d189" distance of L32.end L33.end
  measures "d190" distance of L33.end L34.end
  measures "d191" distance of L34.end L35.end
extrude "Extrude6" [suppressed]
extrude "Extrude7" [suppressed]
hidden bodies 1
equation "lights_length = 264 mm"
equation "lights_width = 32 mm"
equation "lights_depth = 15 mm"
equation "housing_buffer = 20 mm"
equation "mat_thickness = 3 mm"
equation "esp32_length = 57 mm"
equation "esp32_width = 28.5 mm"
equation "button_base_w = 12 mm"
equation "button_d = 5.2 mm"
equation "button_base_depth = 6.5 mm"
equation "button_height = 2 mm"
equation "usb_length = 11 mm"
equation "usb_height = 8 mm"
equation "led_d = 5 mm"
equation "d15 = lights_length"
equation "d16 = lights_width"
equation "d17 = housing_length"
equation "d18 = housing_height"
equation "d19 = clamp_base_width"
equation "d20 = lights_width + 3 * clamp_thick"
equation "d21 = clamp_base_section_height / 2"
equation "d22 = clamp_hole_d"
equation "d23 = clamp_extend_width"
equation "d24 = lights_width + 3 * clamp_thick"
equation "clamp_thick = 2 mm"
equation "led_board_thick = 1.4 mm"
equation "grip_length = 8 mm"
equation "grip_width = 5 mm"
equation "clamp_base_width = 12 mm"
equation "clamp_extend_width = 3 mm"
equation "clamp_hole_d = 3 mm"
equation "d37 = clamp_thick"
equation "led_front_back_thick = 12.5 mm"
equation "d40 = led_front_back_thick - mat_thickness + clamp_thick"
equation "d42 = clamp_thick"
equation "d43 = clamp_thick"
equation "d44 = ( 2 * clamp_thick ) + led_board_thick"
equation "d45 = ( 2 * clamp_thick ) + led_board_thick"
equation "d46 = grip_length + ( clamp_thick * 2 )"
equation "d47 = grip_width"
equation "d49 = clamp_thick"
equation "d50 = clamp_thick"
equation "d51 = grip_length + clamp_thick"
equation "d52 = led_board_thick"
equation "d53 = grip_length + clamp_thick"
equation "d54 = -grip_width"
equation "d56 = -grip_width"
equation "d58 = lights_width / 2"
equation "d63 = clamp_base_width"
equation "d64 = -grip_width"
equation "clamp_base_section_height = 9 mm"
equation "d67 = clamp_base_section_height"
equation "d68 = clamp_base_width"
equation "d69 = clamp_thick"
equation "d71 = lights_length / 2"
equation "d72 = ( lights_width + 3 * clamp_thick ) / 2"
equation "d73 = clamp_extend_width + 1 mm"
equation "d74 = clamp_base_width"
equation "d75 = clamp_base_section_height / 2"
equation "d76 = clamp_hole_d"
equation "d77 = clamp_base_section_height"
equation "d78 = -clamp_extend_width"
equation "housing_length = lights_length + ( 2 * housing_buffer )"
equation "housing_height = lights_width + housing_buffer"
equation "housing_depth = lights_depth + ( 2 * housing_buffer )"
equation "length_fingers = 15"
equation "height_fingers = 3"
equation "depth_fingers = 3"
equation "d86 = mat_thickness"
equation "d87 = ( housing_length / length_fingers ) / 2"
equation "d88 = mat_thickness"
equation "d89 = ( housing_length / length_fingers ) / 2"
equation "d90 = length_fingers"
equation "d92 = housing_length - ( ( housing_length / length_fingers ) )"
equation "d94 = mat_thickness"
equation "d95 = ( housing_length / length_fingers ) / 2"
equation "d96 = mat_thickness"
equation "d97 = ( housing_length / length_fingers ) / 2"
equation "d98 = length_fingers"
equation "d100 = housing_length - ( housing_length / length_fingers )"
equation "length_fingers_measure = ( housing_length / length_fingers ) / 2"
equation "height_fingers_measure = ( housing_height / height_fingers ) / 2"
equation "depth_fingers_measure = ( housing_depth / depth_fingers ) / 2"
equation "d105 = height_fingers_measure"
equation "d106 = mat_thickness"
equation "d107 = height_fingers_measure"
equation "d108 = mat_thickness"
equation "d112 = housing_height - ( height_fingers_measure * 2 )"
equation "d113 = housing_length"
equation "d114 = housing_height"
equation "d115 = housing_height / 2"
equation "d116 = mat_thickness"
equation "d117 = length_fingers_measure"
equation "d118 = mat_thickness"
equation "d119 = length_fingers_measure"
equation "d120 = length_fingers"
equation "d122 = housing_length - ( 2 * length_fingers_measure )"
equation "d124 = length_fingers"
equation "d126 = housing_length - ( 2 * length_fingers_measure )"
equation "d128 = height_fingers_measure"
equation "d129 = mat_thickness"
equation "d130 = height_fingers_measure"
equation "d131 = mat_thickness"
equation "d133 = height_fingers"
equation "d135 = housing_height - ( 2 * height_fingers_measure )"
equation "d137 = height_fingers"
equation "d139 = housing_height - ( 2 * height_fingers_measure )"
equation "d140 = housing_length / 4"
equation "d141 = usb_length"
equation "d142 = usb_height"
equation "esp32_holes_length = 51 mm"
equation "esp32_holes_width = 23 mm"
equation "d145 = esp32_holes_length"
equation "d146 = esp32_holes_width"
equation "d147 = clamp_hole_d"
equation "d148 = housing_length"
equation "d149 = housing_depth"
equation "d150 = length_fingers_measure"
equation "d151 = mat_thickness"
equation "d152 = length_fingers_measure"
equation "d153 = mat_thickness"
equation "d154 = length_fingers"
equation "d156 = housing_length - ( 2 * length_fingers_measure )"
equation "d158 = length_fingers"
equation "d160 = housing_length - ( 2 * length_fingers_measure )"
equation "d162 = mat_thickness"
equation "d163 = depth_fingers_measure"
equation "d164 = mat_thickness"
equation "d165 = depth_fingers_measure"
equation "d167 = depth_fingers"
equation "d169 = housing_depth - ( 2 * depth_fingers_measure )"
equation "d171 = depth_fingers"
equation "d173 = housing_depth - ( 2 * depth_fingers_measure )"
equation "d174 = housing_height"
equation "d175 = housing_depth"
equation "d176 = mat_thickness"
equation "d177 = height_fingers_measure"
equation "d178 = mat_thickness"
equation "d179 = height_fingers_measure"
equation "d180 = height_fingers"
equation "d182 = housing_height - ( 2 * height_fingers_measure )"
equation "d184 = height_fingers"
equation "d186 = housing_height - ( 2 * height_fingers_measure )"
equation "d188 = depth_fingers_measure"
equation "d189 = mat_thickness"
equation "d190 = depth_fingers_measure"
equation "d191 = mat_thickness"
equation "d193 = depth_fingers"
equation "d195 = housing_depth - ( 2 * depth_fingers_measure )"
equation "d197 = depth_fingers"
equation "d199 = housing_depth - ( 2 * depth_fingers_measure )"
named bodies: "Clamps"
